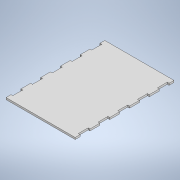
# Autodesk Inventor part: Plate
Saved by Autodesk Inventor 2020 (Build 240168000, 168)
## iProperties
Created: 2019-12-21
Part Number: Plate
Material: Générique
Document SubType Name: Modeling
Designer: damien
Density: 1 g/cm^3
Appearance: Par défaut
Author: damien
Autodesk Inventor part; units mm, degrees
ref_plane "YZ Plane" through (0, 0, 0) normal (1, 0, 0) x (0, 1, 0)
ref_plane "XZ Plane" through (0, 0, 0) normal (0, 1, 0) x (-1, 0, 0)
ref_plane "XY Plane" through (0, 0, 0) normal (0, 0, 1) x (1, 0, 0)
sketch "Esquisse1" plane through (0, 0, 0) normal (0, 1, 0) x (-1, 0, 0)
  line L0 (-350, -500) -> (350, -500)
  line L1 (350, -500) -> (350, 500)
  line L2 (350, 500) -> (-350, 500)
  line L3 (-350, 500) -> (-350, -500)
  line L4 (-350, -500) -> (350, 500) construction
  line L5 (350, -500) -> (-350, 500) construction
  point P0 (0, 0)
  dimension "d0" = 1000
  dimension "d1" = 700
  constraints: 12 end point, 2 midpoint, 2 parallel, 1 horizontal, 1 perpendicular
  measures "d0" distance of L0.end L1.end
  measures "d1" distance of L1.end L2.end
extrude "Extrusion1" add sketch "Esquisse1" along normal blind 18.55
sketch "Esquisse2" plane through (0, 18.55, 0) normal (0, 1, 0) x (1, 0, 0)
  line L0 (-350, 500) -> (-350, -500) projected
  line L1 (-350, -450) -> (-331.45, -450)
  line L2 (-331.45, -450) -> (-331.45, -350)
  line L3 (-331.45, -350) -> (-350, -350)
  line L4 (-350, -350) -> (-350, -450)
  line L5 (-350, -250) -> (-331.45, -250)
  line L6 (-331.45, -250) -> (-331.45, -150)
  line L7 (-331.45, -150) -> (-350, -150)
  line L8 (-350, -150) -> (-350, -250)
  line L9 (-350, -50) -> (-331.45, -50)
  line L10 (-331.45, -50) -> (-331.45, 50)
  line L11 (-331.45, 50) -> (-350, 50)
  line L12 (-350, 50) -> (-350, -50)
  line L13 (-350, 150) -> (-331.45, 150)
  line L14 (-331.45, 150) -> (-331.45, 250)
  line L15 (-331.45, 250) -> (-350, 250)
  line L16 (-350, 250) -> (-350, 150)
  line L17 (350, 500) -> (-350, 500) projected
  line L18 (-350, -500) -> (350, -500) projected
  line L19 (0, -500) -> (0, 500) construction
  line L20 (-350, 350) -> (-331.45, 350)
  line L21 (-331.45, 350) -> (-331.45, 450)
  line L22 (-331.45, 450) -> (-350, 450)
  line L23 (-350, 450) -> (-350, 350)
  line L24 (350, -450) -> (331.45, -450)
  line L25 (331.45, -450) -> (331.45, -350)
  line L26 (331.45, -350) -> (350, -350)
  line L27 (350, -350) -> (350, -450)
  line L28 (350, -250) -> (331.45, -250)
  line L29 (331.45, -250) -> (331.45, -150)
  line L30 (331.45, -150) -> (350, -150)
  line L31 (350, -150) -> (350, -250)
  line L32 (350, -50) -> (331.45, -50)
  line L33 (331.45, -50) -> (331.45, 50)
  line L34 (331.45, 50) -> (350, 50)
  line L35 (350, 50) -> (350, -50)
  line L36 (350, 150) -> (331.45, 150)
  line L37 (331.45, 150) -> (331.45, 250)
  line L38 (331.45, 250) -> (350, 250)
  line L39 (350, 250) -> (350, 150)
  line L40 (350, 350) -> (331.45, 350)
  line L41 (331.45, 350) -> (331.45, 450)
  line L42 (331.45, 450) -> (350, 450)
  line L43 (350, 450) -> (350, 350)
  point P0 (0, 0)
  point P1 (-350, -150)
  point P2 (-350, -250)
  point P3 (-350, 250)
  point P4 (-350, 150)
  point P5 (-350, -350)
  dimension "d6" = 18.55
  dimension "d9" = 200
  dimension "d26" = 50
  dimension "d27" = 100
  dimension "d32" = 50
  constraints: 82 end point, 20 symmetric about line, 2 midpoint, 2 parallel, 1 horizontal, 1 perpendicular, 1 point on line, 1 vertical, 32 other
  measures "d6" distance of L2.end L3.end
  measures "d9" distance of L1.start L5.start
  measures "d26" distance between parallel lines of L18 L1
  measures "d27" distance of L1.end L2.end
  measures "d32" distance between parallel lines of L17 L22
extrude "Extrusion2" cut sketch "Esquisse2" against normal blind 18.55
